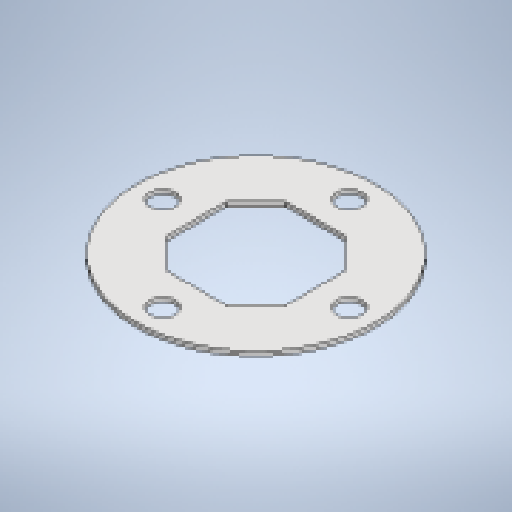
# Autodesk Inventor part: SLM 1651 FDS MAIN  FLANGE
Saved by Autodesk Inventor 2025.3 (Build 293356030, 356C)
## iProperties
Created: 2025-06-24
Part Number: SLM 1651 FDS MAIN  FLANGE
Material: Stainless Steel
Document SubType Name: Sheet Metal
Designer: admin
Mass: 483.479 g
Surface Area: 436.609 cm^2
Volume: 60.4349 cm^3
Density: 8 g/cm^3
Flat Pattern Width: 16 cm
Flat Pattern Length: 16 cm
Flat Pattern Area: 256 cm^2
Sheet Metal Rule: Default
Sheet Metal Width: 160,000 mm
Sheet Metal Length: 160,000 mm
Sheet Metal Area: 25600,000 mm^2
Appearance: Default
Author: user
Autodesk Inventor part; units mm, degrees
ref_plane "YZ Plane" through (0, 0, 0) normal (1, 0, 0) x (0, 1, 0)
ref_plane "XZ Plane" through (0, 0, 0) normal (0, 1, 0) x (-1, 0, 0)
ref_plane "XY Plane" through (0, 0, 0) normal (0, 0, 1) x (1, 0, 0)
sketch "Sketch1" plane through (0, 0, 0) normal (0, 0, 1) x (1, 0, 0)
  circle A0 centre (0, 0) radius 80
  line L0 (40, 40) -> (-40, 40)
  line L1 (-40, 40) -> (-40, -40)
  line L2 (-40, -40) -> (40, -40)
  line L3 (40, -40) -> (40, 40)
  line L4 (40, 40) -> (-40, -40) construction
  line L5 (-40, 40) -> (40, -40) construction
  circle A1 centre (-62.5, 0) radius 8.5
  circle A2 centre (0, 0) radius 62.5 construction
  circle A3 centre (0, -62.5) radius 8.5
  circle A4 centre (62.5, 0) radius 8.5
  circle A5 centre (0, 62.5) radius 8.5
  dimension "d171" = 125
  dimension "d157" = 160
  dimension "d158" = 80
  dimension "d159" = 80
  dimension "d170" = 17
  dimension "d174" = 360
  measures "d157" diameter of A0
  measures "d158" distance of L2.end L1.end
  measures "d159" distance of L1.end L0.end
  measures "d170" diameter of A1
extrude "Plate5" add sketch "Sketch1" along normal blind 3
chamfer "Corner Chamfer2" distance 20 angle 45 4 edges at (-40, -40, 1.5) (40, -40, 1.5) (-40, 40, 1.5) (40, 40, 1.5)
body "Solid3"
